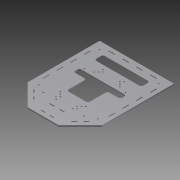
# Autodesk Inventor part: layer 4
Saved by Autodesk Inventor 2012 (Build 160160000, 160)
## iProperties
Created: 2013-01-18
Part Number: layer 4
Material: Default
Document SubType Name: Modeling
Designer: Irwan Haryanto
Density: 1 g/cm^3
Author: Irwan Haryanto
Autodesk Inventor part; units mm, degrees
ref_plane "YZ Plane" through (0, 0, 0) normal (1, 0, 0) x (0, 1, 0)
ref_plane "XZ Plane" through (0, 0, 0) normal (0, 1, 0) x (-1, 0, 0)
ref_plane "XY Plane" through (0, 0, 0) normal (0, 0, 1) x (1, 0, 0)
sketch "Sketch1" plane through (0, 0, 0) normal (0, 0, 1) x (1, 0, 0)
  line L0 (-36.1422, -167.935) -> (36.1422, -167.935)
  line L1 (36.1422, -167.935) -> (87.255, -219.0478)
  line L2 (87.255, -219.0478) -> (87.255, -387.6999)
  line L3 (87.255, -387.6999) -> (-87.255, -387.6999)
  line L4 (-87.255, -387.6999) -> (-87.255, -219.0478)
  line L5 (-87.255, -219.0478) -> (-36.1422, -167.935)
  line L6 (-15.0001, -176.935) -> (-5.0001, -176.935)
  line L7 (-5.0001, -176.935) -> (-5.0001, -178.935)
  line L8 (-5.0001, -178.935) -> (-15.0001, -178.935)
  line L9 (-15.0001, -178.935) -> (-15.0001, -176.935)
  line L10 (5.0001, -178.9353) -> (5.0001, -176.9353)
  line L11 (5.0001, -176.9353) -> (15.0001, -176.9353)
  line L12 (15.0001, -176.9353) -> (15.0001, -178.9353)
  line L13 (15.0001, -178.9353) -> (5.0001, -178.9353)
  line L14 (-57.456, -204.8051) -> (-64.5271, -211.8762)
  line L15 (-65.9413, -210.462) -> (-58.8702, -203.3909)
  line L16 (-64.5271, -211.8762) -> (-65.9413, -210.462)
  line L17 (-58.8702, -203.3909) -> (-57.456, -204.8051)
  line L18 (-44.7279, -189.249) -> (-43.3137, -190.6632)
  line L19 (-43.3137, -190.6632) -> (-50.3848, -197.7342)
  line L20 (-51.799, -196.32) -> (-44.7279, -189.249)
  line L21 (-50.3848, -197.7342) -> (-51.799, -196.32)
  line L22 (57.4002, -204.8577) -> (58.8173, -203.4465)
  line L23 (58.8173, -203.4465) -> (65.8737, -210.5322)
  line L24 (65.8737, -210.5322) -> (64.4565, -211.9435)
  line L25 (64.4565, -211.9435) -> (57.4002, -204.8577)
  line L26 (51.7609, -196.3608) -> (50.3438, -197.772)
  line L27 (43.2874, -190.6863) -> (44.7045, -189.275)
  line L28 (50.3438, -197.772) -> (43.2874, -190.6863)
  line L29 (44.7045, -189.275) -> (51.7609, -196.3608)
  line L30 (-56.4183, -376.6999) -> (-41.4183, -376.6999)
  line L31 (-41.4183, -376.6999) -> (-41.4183, -378.6999)
  line L32 (-41.4183, -378.6999) -> (-56.4183, -378.6999)
  line L33 (-56.4183, -378.6999) -> (-56.4183, -376.6999)
  line L34 (-23.4183, -376.7001) -> (-8.4183, -376.7001)
  line L35 (-8.4183, -376.7001) -> (-8.4183, -378.7001)
  line L36 (-8.4183, -378.7001) -> (-23.4183, -378.7001)
  line L37 (-23.4183, -378.7001) -> (-23.4183, -376.7001)
  line L38 (8.5817, -376.7001) -> (23.5817, -376.7001)
  line L39 (23.5817, -376.7001) -> (23.5817, -378.7001)
  line L40 (23.5817, -378.7001) -> (8.5817, -378.7001)
  line L41 (8.5817, -378.7001) -> (8.5817, -376.7001)
  line L42 (41.5817, -376.7001) -> (56.5817, -376.7001)
  line L43 (56.5817, -376.7001) -> (56.5817, -378.7001)
  line L44 (56.5817, -378.7001) -> (41.5817, -378.7001)
  line L45 (41.5817, -378.7001) -> (41.5817, -376.7001)
  line L46 (-78.255, -341.8632) -> (-76.255, -341.8632)
  line L47 (-76.255, -341.8632) -> (-76.255, -356.8632)
  line L48 (-76.255, -356.8632) -> (-78.255, -356.8632)
  line L49 (-78.255, -356.8632) -> (-78.255, -341.8632)
  line L50 (-78.2548, -308.8632) -> (-76.2548, -308.8632)
  line L51 (-76.2548, -308.8632) -> (-76.2548, -323.8632)
  line L52 (-76.2548, -323.8632) -> (-78.2548, -323.8632)
  line L53 (-78.2548, -323.8632) -> (-78.2548, -308.8632)
  line L54 (-78.2548, -276.8632) -> (-76.2548, -276.8632)
  line L55 (-76.2548, -276.8632) -> (-76.2548, -291.8632)
  line L56 (-76.2548, -291.8632) -> (-78.2548, -291.8632)
  line L57 (-78.2548, -291.8632) -> (-78.2548, -276.8632)
  line L58 (-78.2548, -243.8632) -> (-76.2548, -243.8632)
  line L59 (-76.2548, -243.8632) -> (-76.2548, -258.8632)
  line L60 (-76.2548, -258.8632) -> (-78.2548, -258.8632)
  line L61 (-78.2548, -258.8632) -> (-78.2548, -243.8632)
  line L62 (78.2548, -243.8632) -> (76.2548, -243.8632)
  line L63 (76.2548, -243.8632) -> (76.2548, -258.8632)
  line L64 (76.2548, -258.8632) -> (78.2548, -258.8632)
  line L65 (78.2548, -258.8632) -> (78.2548, -243.8632)
  line L66 (78.2548, -276.8632) -> (76.2548, -276.8632)
  line L67 (76.2548, -291.8632) -> (78.2548, -291.8632)
  line L68 (76.2548, -276.8632) -> (76.2548, -291.8632)
  line L69 (78.2548, -291.8632) -> (78.2548, -276.8632)
  line L70 (76.2548, -308.8632) -> (76.2548, -323.8632)
  line L71 (78.2548, -308.8632) -> (76.2548, -308.8632)
  line L72 (78.2548, -323.8632) -> (78.2548, -308.8632)
  line L73 (76.2548, -323.8632) -> (78.2548, -323.8632)
  line L74 (78.255, -341.8632) -> (76.255, -341.8632)
  line L75 (76.255, -341.8632) -> (76.255, -356.8632)
  line L76 (78.255, -356.8632) -> (78.255, -341.8632)
  line L77 (76.255, -356.8632) -> (78.255, -356.8632)
  line L78 (-16, -202.4164) -> (-16, -200.4164)
  line L79 (-16, -200.4164) -> (-4, -200.4164)
  line L80 (-4, -200.4164) -> (-4, -202.4164)
  line L81 (7, -202.4164) -> (7, -200.4164)
  line L82 (7, -200.4164) -> (19, -200.4164)
  line L83 (19, -200.4164) -> (19, -202.4164)
  line L84 (-20, -247.935) -> (20, -247.935)
  line L85 (25, -252.935) -> (25, -288.735)
  line L86 (20, -307.935) -> (-20, -307.935)
  line L87 (-25, -288.735) -> (-25, -252.935)
  arc A0 (-20, -247.935) -> (-25, -252.935) centre (-20, -252.935) ccw
  arc A1 (25, -252.935) -> (20, -247.935) centre (20, -252.935) ccw
  line L88 (-50, -342.9664) -> (50, -342.9664)
  line L89 (55, -347.9664) -> (55, -357.9664)
  line L90 (50, -362.9664) -> (-50, -362.9664)
  line L91 (-55, -357.9664) -> (-55, -347.9664)
  arc A2 (-50, -342.9664) -> (-55, -347.9664) centre (-50, -347.9664) ccw
  arc A3 (-55, -357.9664) -> (-50, -362.9664) centre (-50, -357.9664) ccw
  arc A4 (50, -362.9664) -> (55, -357.9664) centre (50, -357.9664) ccw
  arc A5 (55, -347.9664) -> (50, -342.9664) centre (50, -347.9664) ccw
  line L92 (30, -293.735) -> (50, -293.735)
  line L93 (55, -298.735) -> (55, -302.935)
  line L94 (50, -307.935) -> (20, -307.935)
  line L95 (-30, -293.735) -> (-50, -293.735)
  line L96 (-55, -298.735) -> (-55, -302.935)
  line L97 (-50, -307.935) -> (-20, -307.935)
  arc A6 (-30, -293.735) -> (-25, -288.735) centre (-30, -288.735) ccw
  arc A7 (-50, -293.735) -> (-55, -298.735) centre (-50, -298.735) ccw
  arc A8 (-55, -302.935) -> (-50, -307.935) centre (-50, -302.935) ccw
  arc A9 (50, -307.935) -> (55, -302.935) centre (50, -302.935) ccw
  arc A10 (55, -298.735) -> (50, -293.735) centre (50, -298.735) ccw
  arc A11 (25, -288.735) -> (30, -293.735) centre (30, -288.735) ccw
  line L98 (-16, -202.4164) -> (-4, -202.4164)
  line L99 (7, -202.4164) -> (19, -202.4164)
  point P0 (-39.3214, -278.2062)
  point P1 (25, -307.935)
  point P2 (-25, -307.935)
  point P3 (-55, -342.9664)
  point P4 (55, -362.9664)
  point P5 (55, -342.9664)
  point P6 (25, -293.735)
  point P7 (55, -293.735)
  point P8 (-25, -293.735)
  point P9 (-55, -293.735)
  dimension "d12" = 10
  dimension "d13" = 2
  dimension "d16" = 10
  dimension "d17" = 2
  dimension "d19" = 10
  dimension "d20" = 2
  dimension "d23" = 10
  dimension "d24" = 2
  dimension "d25" = 10
  dimension "d26" = 10
  dimension "d27" = 2
  dimension "d28" = 10
  dimension "d29" = 2
  dimension "d30" = 10
  dimension "d33" = 15
  dimension "d34" = 2
  dimension "d36" = 15
  dimension "d37" = 18
  dimension "d38" = 15
  dimension "d39" = 17
  dimension "d40" = 2
  dimension "d41" = 15
  dimension "d43" = 15
  dimension "d44" = 18
  dimension "d45" = 15
  dimension "d46" = 17
  dimension "d47" = 15
  dimension "d48" = 18
  dimension "d52" = 15
  dimension "d54" = 18
  dimension "d55" = 219.7649
  dimension "d56" = 174.51
  dimension "d112" = 2
  dimension "d113" = 12
  dimension "d114" = 12
  dimension "d116" = 11
  dimension "d208" = 50
  dimension "d211" = 60
  dimension "d212" = 5
  dimension "d213" = 110
  dimension "d214" = 20
  dimension "d217" = 5
  dimension "d254" = 30
  dimension "d255" = 30
  dimension "d256" = 5
  constraints: 200 end point, 36 parallel, 27 perpendicular, 24 point on circle, 24 tangent, 18 point on line, 12 centre point, 12 horizontal, 9 equal radius
  measures "d12" distance of L7.end L8.end
  measures "d13" distance of L6.end L7.end
  measures "d16" distance of L12.end L10.start
  measures "d17" distance of L11.end L12.end
  measures "d19" distance of L14.start L14.end
  measures "d20" distance of L15.end L14.start
  measures "d23" distance of L18.end L19.end
  measures "d24" distance of L18.start L18.end
  measures "d25" distance between parallel lines of L21 L17
  measures "d26" distance of L26.end L27.start
  measures "d27" distance of L26.start L26.end
  measures "d28" distance of L24.end L22.start
  measures "d29" distance of L23.end L24.end
  measures "d30" distance between parallel lines of L22 L26
  measures "d33" distance of L31.end L32.end
  measures "d34" distance of L30.end L31.end
  measures "d36" distance of L35.end L36.end
  measures "d37" distance between parallel lines of L37 L31
  measures "d38" distance of L39.end L40.end
  measures "d39" distance between parallel lines of L41 L35
  measures "d40" distance of L47.end L48.end
  measures "d41" distance of L46.end L47.end
  measures "d43" distance of L50.end L51.end
  measures "d44" distance between parallel lines of L46 L52
  measures "d45" distance of L54.end L55.end
  measures "d46" distance between parallel lines of L50 L56
  measures "d47" distance of L58.end L59.end
  measures "d48" distance between parallel lines of L60 L54
  measures "d52" distance between parallel lines of L43 L45
  measures "d54" distance between parallel lines of L45 L39
  measures "d55" distance between parallel lines of L3 L0
  measures "d56" distance between parallel lines of L2 L4
  measures "d112" distance of L78.start L78.end
  measures "d113" distance of L78.end L79.end
  measures "d114" distance of L81.end L82.end
  measures "d116" distance between parallel lines of L81 L80
  measures "d208" distance of point (25, -307.935) point (-25, -307.935)
  measures "d211" distance between parallel lines of L86 L84
  measures "d212" radius of A0
  measures "d213" distance of point (-55, -342.966) point (55, -342.966)
  measures "d214" distance of point (55, -342.966) point (55, -362.966)
  measures "d217" radius of A2
  measures "d254" distance of point (-25, -293.735) point (-55, -293.735)
  measures "d255" distance of point (25, -293.735) point (55, -293.735)
  measures "d256" radius of A6
extrude "Extrusion1" add sketch "Sketch1" along normal blind 3
sketch "Sketch2" plane through (0, 0, 3) normal (0, 0, 1) x (1, 0, 0)
  line L0 (-36.1422, -167.935) -> (36.1422, -167.935)
  line L1 (36.1422, -167.935) -> (87.255, -219.0478)
  line L2 (87.255, -219.0478) -> (87.255, -387.6999)
  line L3 (87.255, -387.6999) -> (-87.255, -387.6999)
  line L4 (-87.255, -387.6999) -> (-87.255, -219.0478)
  line L5 (-87.255, -219.0478) -> (-36.1422, -167.935)
  line L6 (-15.0001, -176.935) -> (-5.0001, -176.935)
  line L7 (-5.0001, -176.935) -> (-5.0001, -178.935)
  line L8 (-5.0001, -178.935) -> (-15.0001, -178.935)
  line L9 (-15.0001, -178.935) -> (-15.0001, -176.935)
  line L10 (5.0001, -178.9353) -> (5.0001, -176.9353)
  line L11 (5.0001, -176.9353) -> (15.0001, -176.9353)
  line L12 (15.0001, -176.9353) -> (15.0001, -178.9353)
  line L13 (15.0001, -178.9353) -> (5.0001, -178.9353)
  line L14 (-57.456, -204.8051) -> (-64.5271, -211.8762)
  line L15 (-65.9413, -210.462) -> (-58.8702, -203.3909)
  line L16 (-64.5271, -211.8762) -> (-65.9413, -210.462)
  line L17 (-58.8702, -203.3909) -> (-57.456, -204.8051)
  line L18 (-44.7279, -189.249) -> (-43.3137, -190.6632)
  line L19 (-43.3137, -190.6632) -> (-50.3848, -197.7342)
  line L20 (-51.799, -196.32) -> (-44.7279, -189.249)
  line L21 (-50.3848, -197.7342) -> (-51.799, -196.32)
  line L22 (57.4002, -204.8577) -> (58.8173, -203.4465)
  line L23 (58.8173, -203.4465) -> (65.8737, -210.5322)
  line L24 (65.8737, -210.5322) -> (64.4565, -211.9435)
  line L25 (64.4565, -211.9435) -> (57.4002, -204.8577)
  line L26 (51.7609, -196.3608) -> (50.3438, -197.772)
  line L27 (43.2874, -190.6863) -> (44.7045, -189.275)
  line L28 (50.3438, -197.772) -> (43.2874, -190.6863)
  line L29 (44.7045, -189.275) -> (51.7609, -196.3608)
  line L30 (-56.4183, -376.6999) -> (-41.4183, -376.6999)
  line L31 (-41.4183, -376.6999) -> (-41.4183, -378.6999)
  line L32 (-41.4183, -378.6999) -> (-56.4183, -378.6999)
  line L33 (-56.4183, -378.6999) -> (-56.4183, -376.6999)
  line L34 (-23.4183, -376.7001) -> (-8.4183, -376.7001)
  line L35 (-8.4183, -376.7001) -> (-8.4183, -378.7001)
  line L36 (-8.4183, -378.7001) -> (-23.4183, -378.7001)
  line L37 (-23.4183, -378.7001) -> (-23.4183, -376.7001)
  line L38 (8.5817, -376.7001) -> (23.5817, -376.7001)
  line L39 (23.5817, -376.7001) -> (23.5817, -378.7001)
  line L40 (23.5817, -378.7001) -> (8.5817, -378.7001)
  line L41 (8.5817, -378.7001) -> (8.5817, -376.7001)
  line L42 (41.5817, -376.7001) -> (56.5817, -376.7001)
  line L43 (56.5817, -376.7001) -> (56.5817, -378.7001)
  line L44 (56.5817, -378.7001) -> (41.5817, -378.7001)
  line L45 (41.5817, -378.7001) -> (41.5817, -376.7001)
  line L46 (-78.255, -341.8632) -> (-76.255, -341.8632)
  line L47 (-76.255, -341.8632) -> (-76.255, -356.8632)
  line L48 (-76.255, -356.8632) -> (-78.255, -356.8632)
  line L49 (-78.255, -356.8632) -> (-78.255, -341.8632)
  line L50 (-78.2548, -308.8632) -> (-76.2548, -308.8632)
  line L51 (-76.2548, -308.8632) -> (-76.2548, -323.8632)
  line L52 (-76.2548, -323.8632) -> (-78.2548, -323.8632)
  line L53 (-78.2548, -323.8632) -> (-78.2548, -308.8632)
  line L54 (-78.2548, -276.8632) -> (-76.2548, -276.8632)
  line L55 (-76.2548, -276.8632) -> (-76.2548, -291.8632)
  line L56 (-76.2548, -291.8632) -> (-78.2548, -291.8632)
  line L57 (-78.2548, -291.8632) -> (-78.2548, -276.8632)
  line L58 (-78.2548, -243.8632) -> (-76.2548, -243.8632)
  line L59 (-76.2548, -243.8632) -> (-76.2548, -258.8632)
  line L60 (-76.2548, -258.8632) -> (-78.2548, -258.8632)
  line L61 (-78.2548, -258.8632) -> (-78.2548, -243.8632)
  line L62 (78.2548, -243.8632) -> (76.2548, -243.8632)
  line L63 (76.2548, -243.8632) -> (76.2548, -258.8632)
  line L64 (76.2548, -258.8632) -> (78.2548, -258.8632)
  line L65 (78.2548, -258.8632) -> (78.2548, -243.8632)
  line L66 (78.2548, -276.8632) -> (76.2548, -276.8632)
  line L67 (76.2548, -291.8632) -> (78.2548, -291.8632)
  line L68 (76.2548, -276.8632) -> (76.2548, -291.8632)
  line L69 (78.2548, -291.8632) -> (78.2548, -276.8632)
  line L70 (76.2548, -308.8632) -> (76.2548, -323.8632)
  line L71 (78.2548, -308.8632) -> (76.2548, -308.8632)
  line L72 (78.2548, -323.8632) -> (78.2548, -308.8632)
  line L73 (76.2548, -323.8632) -> (78.2548, -323.8632)
  line L74 (78.255, -341.8632) -> (76.255, -341.8632)
  line L75 (76.255, -341.8632) -> (76.255, -356.8632)
  line L76 (78.255, -356.8632) -> (78.255, -341.8632)
  line L77 (76.255, -356.8632) -> (78.255, -356.8632)
  circle A0 centre (19.4208, -227.9164) radius 1.5
  circle A1 centre (19.4208, -217.9164) radius 1.5
  circle A2 centre (24.975, -232.9164) radius 1.5
  circle A3 centre (29.975, -238.0334) radius 1.5
  circle A4 centre (24.975, -222.9164) radius 1.5
  circle A5 centre (-29.975, -238.0334) radius 1.5
  circle A6 centre (-19.4208, -227.9164) radius 1.5
  circle A7 centre (-24.975, -222.9164) radius 1.5
  circle A8 centre (-19.4208, -217.9164) radius 1.5
  circle A9 centre (-24.975, -232.9164) radius 1.5
  circle A10 centre (24.975, -322.9664) radius 1.5
  circle A11 centre (29.975, -317.8494) radius 1.5
  circle A12 centre (19.975, -327.9664) radius 1.5
  circle A13 centre (24.975, -332.9664) radius 1.5
  circle A14 centre (-19.975, -327.9664) radius 1.5
  circle A15 centre (-24.975, -322.9664) radius 1.5
  circle A16 centre (-29.975, -317.8494) radius 1.5
  circle A17 centre (-24.975, -332.9664) radius 1.5
  line L78 (-16, -202.4164) -> (-16, -200.4164)
  line L79 (-16, -200.4164) -> (-4, -200.4164)
  line L80 (-4, -200.4164) -> (-4, -202.4164)
  line L81 (7, -202.4164) -> (7, -200.4164)
  line L82 (7, -200.4164) -> (19, -200.4164)
  line L83 (19, -200.4164) -> (19, -202.4164)
  circle A18 centre (69.255, -226.5036) radius 1.5
  circle A19 centre (-69.255, -226.5036) radius 1.5
  circle A20 centre (69.255, -369.6999) radius 1.5
  circle A21 centre (-69.255, -369.6999) radius 1.5
  circle A22 centre (48, -312.935) radius 1.5
  circle A23 centre (-47.9336, -312.935) radius 1.5
  circle A24 centre (-47.9336, -216.435) radius 1.5
  circle A25 centre (48, -216.435) radius 1.5
  line L84 (-20, -247.935) -> (20, -247.935)
  line L85 (25, -252.935) -> (25, -288.735)
  line L86 (20, -307.935) -> (-20, -307.935)
  line L87 (-25, -288.735) -> (-25, -252.935)
  arc A26 (-20, -247.935) -> (-25, -252.935) centre (-20, -252.935) ccw
  arc A27 (25, -252.935) -> (20, -247.935) centre (20, -252.935) ccw
  line L88 (-50, -342.9664) -> (50, -342.9664)
  line L89 (55, -347.9664) -> (55, -357.9664)
  line L90 (50, -362.9664) -> (-50, -362.9664)
  line L91 (-55, -357.9664) -> (-55, -347.9664)
  arc A28 (-50, -342.9664) -> (-55, -347.9664) centre (-50, -347.9664) ccw
  arc A29 (-55, -357.9664) -> (-50, -362.9664) centre (-50, -357.9664) ccw
  arc A30 (50, -362.9664) -> (55, -357.9664) centre (50, -357.9664) ccw
  arc A31 (55, -347.9664) -> (50, -342.9664) centre (50, -347.9664) ccw
  line L92 (30, -293.735) -> (50, -293.735)
  line L93 (55, -298.735) -> (55, -302.935)
  line L94 (50, -307.935) -> (20, -307.935)
  line L95 (-30, -293.735) -> (-50, -293.735)
  line L96 (-55, -298.735) -> (-55, -302.935)
  line L97 (-50, -307.935) -> (-20, -307.935)
  arc A32 (-30, -293.735) -> (-25, -288.735) centre (-30, -288.735) ccw
  arc A33 (-50, -293.735) -> (-55, -298.735) centre (-50, -298.735) ccw
  arc A34 (-55, -302.935) -> (-50, -307.935) centre (-50, -302.935) ccw
  arc A35 (50, -307.935) -> (55, -302.935) centre (50, -302.935) ccw
  arc A36 (55, -298.735) -> (50, -293.735) centre (50, -298.735) ccw
  arc A37 (25, -288.735) -> (30, -293.735) centre (30, -288.735) ccw
  line L98 (-16, -202.4164) -> (-4, -202.4164)
  line L99 (7, -202.4164) -> (19, -202.4164)
  point P0 (0, 0)
  point P1 (-39.3214, -278.2062)
  point P2 (25, -307.935)
  point P3 (-25, -307.935)
  point P4 (25, -293.735)
  point P5 (-25, -293.735)
  point P6 (-55, -342.9664)
  point P7 (55, -362.9664)
  point P8 (55, -342.9664)
  point P9 (55, -293.735)
  point P10 (-55, -293.735)
  dimension "d259" = 10
  dimension "d260" = 2
  dimension "d261" = 10
  dimension "d262" = 2
  dimension "d263" = 10
  dimension "d264" = 2
  dimension "d265" = 10
  dimension "d266" = 2
  dimension "d267" = 10
  dimension "d268" = 10
  dimension "d269" = 2
  dimension "d270" = 10
  dimension "d271" = 2
  dimension "d272" = 10
  dimension "d273" = 15
  dimension "d274" = 2
  dimension "d275" = 15
  dimension "d276" = 18
  dimension "d277" = 15
  dimension "d278" = 17
  dimension "d279" = 2
  dimension "d280" = 15
  dimension "d281" = 15
  dimension "d282" = 18
  dimension "d283" = 15
  dimension "d284" = 17
  dimension "d285" = 15
  dimension "d286" = 18
  dimension "d287" = 15
  dimension "d288" = 18
  dimension "d289" = 219.7649
  dimension "d290" = 174.51
  dimension "d291" = 3
  dimension "d292" = 3
  dimension "d293" = 3
  dimension "d294" = 3
  dimension "d295" = 3
  dimension "d296" = -5.117
  dimension "d297" = 10
  dimension "d298" = 15.117
  dimension "d299" = 10
  dimension "d300" = 5.5542
  dimension "d301" = 5
  dimension "d302" = 5
  dimension "d303" = 5.5542
  dimension "d304" = 5.5542
  dimension "d305" = 5
  dimension "d306" = 5
  dimension "d307" = 3
  dimension "d308" = 3
  dimension "d309" = 3
  dimension "d310" = 5.117
  dimension "d311" = 0
  dimension "d312" = 15.117
  dimension "d313" = 3
  dimension "d314" = 5
  dimension "d315" = 5
  dimension "d316" = 5
  dimension "d317" = 5
  dimension "d318" = 5
  dimension "d319" = 2
  dimension "d320" = 12
  dimension "d321" = 12
  dimension "d322" = 11
  constraints: 200 end point, 38 centre point, 36 parallel, 27 perpendicular, 24 point on circle, 24 tangent, 18 point on line, 12 horizontal, 9 equal radius
  measures "d259" distance of L7.end L8.end
  measures "d260" distance of L7.start L7.end
  measures "d261" distance of L13.start L13.end
  measures "d262" distance of L12.start L13.start
  measures "d263" distance of L14.start L14.end
  measures "d264" distance of L15.end L14.start
  measures "d265" distance of L19.start L21.start
  measures "d266" distance of L18.start L19.start
  measures "d267" distance between parallel lines of L21 L17
  measures "d268" distance of L26.end L28.end
  measures "d269" distance of L26.start L26.end
  measures "d270" distance of L25.start L25.end
  measures "d271" distance of L23.end L25.start
  measures "d272" distance between parallel lines of L22 L26
  measures "d273" distance of L32.start L33.start
  measures "d274" distance of L30.end L32.start
  measures "d275" distance of L35.end L36.end
  measures "d276" distance between parallel lines of L37 L31
  measures "d277" distance of L39.end L40.end
  measures "d278" distance between parallel lines of L41 L35
  measures "d279" distance of L48.start L48.end
  measures "d280" distance of L47.start L48.start
  measures "d281" distance of L51.start L52.start
  measures "d282" distance between parallel lines of L46 L52
  measures "d283" distance of L54.end L55.end
  measures "d284" distance between parallel lines of L50 L56
  measures "d285" distance of L58.end L59.end
  measures "d286" distance between parallel lines of L60 L54
  measures "d287" distance between parallel lines of L43 L45
  measures "d288" distance between parallel lines of L45 L39
  measures "d289" distance between parallel lines of L3 L0
  measures "d290" distance between parallel lines of L2 L4
  measures "d291" diameter of A3
  measures "d292" diameter of A2
  measures "d293" diameter of A4
  measures "d294" diameter of A0
  measures "d295" diameter of A1
  measures "d296" vertical distance of A2.centre A3.centre
  measures "d297" distance of A2.centre A4.centre
  measures "d298" vertical distance of A3.centre A4.centre
  measures "d299" distance of A0.centre A1.centre
  measures "d300" horizontal distance of A0.centre A4.centre
  measures "d301" vertical distance of A4.centre A1.centre
  measures "d302" vertical distance of A0.centre A4.centre
  measures "d303" horizontal distance of A4.centre A1.centre
  measures "d304" horizontal distance of A2.centre A0.centre
  measures "d305" vertical distance of A2.centre A0.centre
  measures "d306" horizontal distance of A3.centre A2.centre
  measures "d307" diameter of A10
  measures "d308" diameter of A13
  measures "d309" diameter of A11
  measures "d310" vertical distance of A10.centre A11.centre
  measures "d311" horizontal distance of A13.centre A10.centre
  measures "d312" vertical distance of A13.centre A11.centre
  measures "d313" diameter of A12
  measures "d314" horizontal distance of A12.centre A10.centre
  measures "d315" horizontal distance of A12.centre A10.centre
  measures "d316" horizontal distance of A12.centre A13.centre
  measures "d317" horizontal distance of A13.centre A12.centre
  measures "d318" horizontal distance of A10.centre A11.centre
  measures "d319" distance of L98.start L79.start
  measures "d320" distance of L79.start L80.start
  measures "d321" distance of L81.end L82.end
  measures "d322" distance between parallel lines of L81 L80
hole "Hole1" at (-69.255, -226.5036, 3) at (-47.9336, -216.435, 3) at (-19.4208, -217.9164, 3) at (-24.975, -222.9164, 3) at (-19.4208, -227.9164, 3) at (-24.975, -232.9164, 3) at (-29.975, -238.0334, 3) at (19.4208, -217.9164, 3) at (24.975, -222.9164, 3) at (19.4208, -227.9164, 3) at (24.975, -232.9164, 3) at (29.975, -238.0334, 3) at (48, -216.435, 3) at (69.255, -226.5036, 3) at (48, -312.935, 3) at (29.975, -317.8494, 3) at (24.975, -322.9664, 3) at (19.975, -327.9664, 3) at (24.975, -332.9664, 3) at (-47.9336, -312.935, 3) at (-29.975, -317.8494, 3) at (-24.975, -322.9664, 3) at (-19.975, -327.9664, 3) at (-24.975, -332.9664, 3) at (-69.255, -369.6999, 3) at (69.255, -369.6999, 3) direction (0, 0, -1) diameter 3 end through all
body "Solid1"
